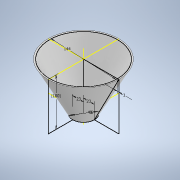
# Autodesk Inventor part: cone
Saved by Autodesk Inventor 2020 (Build 240168000, 168)
## iProperties
Created: 2020-12-15
Part Number: cone
Material: Generic
Document SubType Name: Modeling
Designer: moham
Density: 1 g/cm^3
Appearance: Default
Author: moham
Autodesk Inventor part; units mm, degrees
ref_plane "YZ Plane" through (0, 0, 0) normal (1, 0, 0) x (0, 1, 0)
ref_plane "XZ Plane" through (0, 0, 0) normal (0, 1, 0) x (-1, 0, 0)
ref_plane "XY Plane" through (0, 0, 0) normal (0, 0, 1) x (1, 0, 0)
sketch "Sketch1" plane through (0, 0, 0) normal (0, 1, 0) x (-1, 0, 0)
  circle A0 centre (0, 0) radius 75
  dimension "d0" = 150
  constraints: 1 centre point, 1 coincident
  measures "d0" diameter of A0
extrude "Extrusion1" add sketch "Sketch1" against normal blind 100
sketch "Sketch2" plane through (0, 0, 0) normal (0, 1, 0) x (1, 0, 0)
  circle A0 centre (0, 0) radius 72
  dimension "d3" = 144
  constraints: 1 centre point, 1 coincident
  measures "d3" diameter of A0
sketch "Sketch4" plane through (0, 0, 0) normal (0, 0, 1) x (1, 0, 0)
  line L0 (-75, -100) -> (75, -100) projected
  line L1 (0, -100) -> (23, -100)
  line L2 (75, 0) -> (-75, 0) projected
  line L3 (23, -100) -> (75, 0)
  line L4 (75, 0) -> (23, -100)
  line L5 (23, -100) -> (75, 0)
  line L6 (75, 0) -> (23, -100)
  line L7 (0, -100) -> (-23, -100)
  line L8 (-75, 0) -> (-23, -100)
  line L9 (75, 0) -> (75, -100)
  line L10 (23, -100) -> (75, -100)
  line L11 (0, -120) -> (0, 20) projected
  line L12 (75, 0) -> (72, 0)
  line L13 (72, 0) -> (20, -100)
  line L14 (20, -100) -> (0, -100)
  line L15 (0, -100) -> (0, 0)
  line L16 (0, 0) -> (72, 0)
  dimension "d5" = 23
  dimension "d10" = 23
  dimension "d14" = 3
  constraints: 28 end point, 7 collinear, 4 point on line, 1 midpoint, 1 parallel, 1 vertical
  measures "d5" distance of L1.start L1.end
  measures "d10" distance of L1.start L7.end
  measures "d14" distance of L2.start L12.end
sketch "Sketch7" plane through (0, 0, 0) normal (1, 0, 0) x (0, 1, 0)
  line L0 (0, -75) -> (0, 75) projected
  line L1 (0, 75) -> (-100, 75)
  line L2 (0, 75) -> (-100, 75) projected
  line L3 (-100, 75) -> (-100, -75) projected
  line L4 (-100, 75) -> (-100, 20)
  point P0 (0, 0)
  dimension "d9" = 100
  constraints: 4 end point, 2 point on line
  measures "d9" distance of L0.end L1.end
sketch "Sketch11" plane through (0, -100, 0) normal (0, -1, 0) x (1, 0, 0)
  circle A0 centre (0, 0) radius 20
  circle A1 centre (0, 0) radius 23
  dimension "d11" = 40
  dimension "d12" = 46
  constraints: 2 centre point, 2 coincident
  measures "d11" diameter of A0
  measures "d12" diameter of A1
revolve "Revolution3" cut sketch "Sketch4" angle 360 about axis through (0, -10, 0) along (0, 1, 0) contours L3 L9 L0
revolve "Revolution4" cut sketch "Sketch4" angle 360 about axis through (0, -10, 0) along (0, 1, 0) contours L11 L2 L13 L0
body "Solid1"
